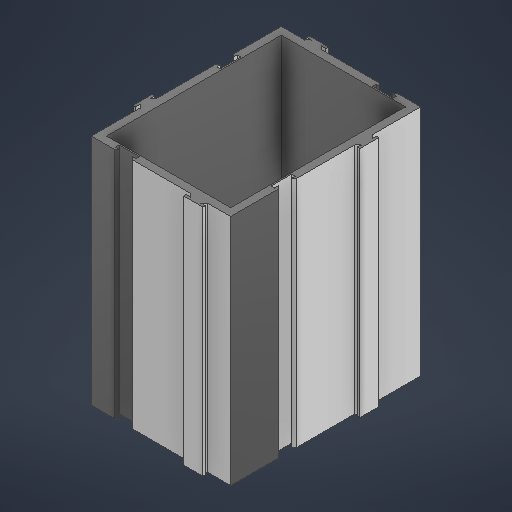
# Autodesk Inventor part: box
Saved by Autodesk Inventor 2027 (Build 310192060, 192F)
## iProperties
Created: 2026-06-08
Part Number: box
Material: Ogólny
Document SubType Name: Modeling
Designer: User
Density: 1 g/cm^3
Appearance: Domyślna
Author: User
Autodesk Inventor part; units mm, degrees
ref_plane "YZ Plane" through (0, 0, 0) normal (1, 0, 0) x (0, 1, 0)
ref_plane "XZ Plane" through (0, 0, 0) normal (0, 1, 0) x (-1, 0, 0)
ref_plane "XY Plane" through (0, 0, 0) normal (0, 0, 1) x (1, 0, 0)
sketch "Szkic1" plane through (0, 0, 0) normal (0, 1, 0) x (-1, 0, 0)
  line L0 (-27.5, -37.5) -> (27.5, -37.5)
  line L1 (27.5, -37.5) -> (27.5, 37.5)
  line L2 (27.5, 37.5) -> (-27.5, 37.5)
  line L3 (-27.5, 37.5) -> (-27.5, -37.5)
  line L4 (-27.5, -37.5) -> (27.5, 37.5) construction
  line L5 (27.5, -37.5) -> (-27.5, 37.5) construction
  line L6 (-24.5, -34.5) -> (24.5, -34.5)
  line L7 (24.5, -34.5) -> (24.5, 34.5)
  line L8 (24.5, 34.5) -> (-24.5, 34.5)
  line L9 (-24.5, 34.5) -> (-24.5, -34.5)
  line L10 (-24.5, -34.5) -> (24.5, 34.5) construction
  line L11 (24.5, -34.5) -> (-24.5, 34.5) construction
  line L12 (27.5, 37.5) -> (18.5607, 37.5)
  line L13 (27.5, 37.5) -> (36.4393, 37.5) construction
  line L14 (18.5607, 37.5) -> (17.5, 36.4393)
  line L15 (17.5, 36.4393) -> (19, 36.4393)
  line L16 (19, 36.4393) -> (19, 35.0393)
  line L17 (-27.5, 37.5) -> (-25.5, 37.5) construction
  line L18 (0, 34.5) -> (0, 37.5) construction
  line L19 (18.5607, 37.5) -> (32.6482, 37.5) construction
  line L20 (11.4393, 37.5) -> (29.6482, 37.5) construction
  line L21 (19, 35.0393) -> (15, 35.0393)
  line L22 (15, 35.0393) -> (15, 37.5) construction
  line L23 (11.4393, 37.5) -> (12.5, 36.4393)
  line L24 (12.5, 36.4393) -> (11, 36.4393)
  line L25 (11, 36.4393) -> (11, 35.0393)
  line L26 (11, 35.0393) -> (15, 35.0393)
  line L27 (-18.5607, 37.5) -> (-17.5, 36.4393) construction
  line L28 (-17.5, 36.4393) -> (-19, 36.4393) construction
  line L29 (-19, 35.0393) -> (-15, 35.0393) construction
  line L30 (-15, 35.0393) -> (-15, 37.5) construction
  line L31 (-11.4393, 37.5) -> (-12.5, 36.4393) construction
  line L32 (-11, 35.0393) -> (-15, 35.0393) construction
  line L33 (-11, 36.4393) -> (-11, 35.0393) construction
  line L34 (-12.5, 36.4393) -> (-11, 36.4393) construction
  line L35 (-19, 36.4393) -> (-19, 35.0393) construction
  line L36 (24.5, 0) -> (-24.5, 0) construction
  line L37 (27.5, 0) -> (24.5, 0) construction
  line L38 (18.5607, -37.5) -> (17.5, -36.4393) construction
  line L39 (17.5, -36.4393) -> (19, -36.4393) construction
  line L40 (19, -36.4393) -> (19, -35.0393) construction
  line L41 (19, -35.0393) -> (15, -35.0393) construction
  line L42 (15, -35.0393) -> (15, -37.5) construction
  line L43 (11.4393, -37.5) -> (12.5, -36.4393) construction
  line L44 (11, -35.0393) -> (15, -35.0393) construction
  line L45 (11, -36.4393) -> (11, -35.0393) construction
  line L46 (12.5, -36.4393) -> (11, -36.4393) construction
  line L47 (-11.4393, -37.5) -> (-12.5, -36.4393)
  line L48 (-12.5, -36.4393) -> (-11, -36.4393)
  line L49 (-15, -35.0393) -> (-15, -37.5) construction
  line L50 (-11, -35.0393) -> (-15, -35.0393)
  line L51 (-18.5607, -37.5) -> (-17.5, -36.4393)
  line L52 (-17.5, -36.4393) -> (-19, -36.4393)
  line L53 (-19, -35.0393) -> (-15, -35.0393)
  line L54 (-11, -36.4393) -> (-11, -35.0393)
  line L55 (-19, -36.4393) -> (-19, -35.0393)
  line L56 (27.5, 11.4393) -> (26.4393, 12.5) construction
  line L57 (26.4393, 12.5) -> (26.4393, 11) construction
  line L58 (26.4393, 11) -> (25.0393, 11) construction
  line L59 (25.0393, 11) -> (25.0393, 15) construction
  line L60 (25.0393, 15) -> (27.3, 15) construction
  line L61 (27.5, 18.5607) -> (26.4393, 17.5) construction
  line L62 (25.0393, 19) -> (25.0393, 15) construction
  line L63 (26.4393, 19) -> (25.0393, 19) construction
  line L64 (26.4393, 17.5) -> (26.4393, 19) construction
  line L65 (27.5, -11.4393) -> (26.4393, -12.5)
  line L66 (26.4393, -12.5) -> (26.4393, -11)
  line L67 (26.4393, -11) -> (25.0393, -11)
  line L68 (25.0393, -11) -> (25.0393, -15)
  line L69 (27.5, -18.5607) -> (26.4393, -17.5)
  line L70 (26.4393, -17.5) -> (26.4393, -19)
  line L71 (25.0393, -15) -> (27.3, -15) construction
  line L72 (25.0393, -19) -> (25.0393, -15)
  line L73 (26.4393, -19) -> (25.0393, -19)
  line L74 (-27.5, 11.4393) -> (-26.4393, 12.5)
  line L75 (-26.4393, 12.5) -> (-26.4393, 11)
  line L76 (-26.4393, 11) -> (-25.0393, 11)
  line L77 (-25.0393, 11) -> (-25.0393, 15)
  line L78 (-27.5, 18.5607) -> (-26.4393, 17.5)
  line L79 (-26.4393, 17.5) -> (-26.4393, 19)
  line L80 (-25.0393, 15) -> (-27.3, 15) construction
  line L81 (-25.0393, 19) -> (-25.0393, 15)
  line L82 (-26.4393, 19) -> (-25.0393, 19)
  line L83 (-27.5, -11.4393) -> (-26.4393, -12.5) construction
  line L84 (-26.4393, -12.5) -> (-26.4393, -11) construction
  line L85 (-26.4393, -11) -> (-25.0393, -11) construction
  line L86 (-25.0393, -11) -> (-25.0393, -15) construction
  line L87 (-25.0393, -15) -> (-27.3, -15) construction
  line L88 (-27.5, -18.5607) -> (-26.4393, -17.5) construction
  line L89 (-25.0393, -19) -> (-25.0393, -15) construction
  line L90 (-26.4393, -17.5) -> (-26.4393, -19) construction
  line L91 (-26.4393, -19) -> (-25.0393, -19) construction
  line L92 (-11.4393, 37.5) -> (-12.5, 38.5607)
  line L93 (-12.5, 38.5607) -> (-11, 38.5607)
  line L94 (-15, 39.9607) -> (-15, 37.5)
  line L95 (-11, 39.9607) -> (-15, 39.9607)
  line L96 (-18.5607, 37.5) -> (-17.5, 38.5607)
  line L97 (-17.5, 38.5607) -> (-19, 38.5607)
  line L98 (-19, 39.9607) -> (-15, 39.9607)
  line L99 (-11, 38.5607) -> (-11, 39.9607)
  line L100 (-19, 38.5607) -> (-19, 39.9607)
  line L101 (18.5607, -37.5) -> (17.5, -38.5607)
  line L102 (17.5, -38.5607) -> (19, -38.5607)
  line L103 (19, -38.5607) -> (19, -39.9607)
  line L104 (19, -39.9607) -> (15, -39.9607)
  line L105 (11, -39.9607) -> (15, -39.9607)
  line L106 (15, -39.9607) -> (15, -37.5) construction
  line L107 (11.4393, -37.5) -> (12.5, -38.5607)
  line L108 (11, -38.5607) -> (11, -39.9607)
  line L109 (12.5, -38.5607) -> (11, -38.5607)
  line L110 (27.5, 11.4393) -> (28.5607, 12.5)
  line L111 (28.5607, 12.5) -> (28.5607, 11)
  line L112 (28.5607, 11) -> (29.9607, 11)
  line L113 (29.9607, 11) -> (29.9607, 15)
  line L114 (27.5, 18.5607) -> (28.5607, 17.5)
  line L115 (28.5607, 17.5) -> (28.5607, 19)
  line L116 (29.9607, 15) -> (27.7, 15) construction
  line L117 (29.9607, 19) -> (29.9607, 15)
  line L118 (28.5607, 19) -> (29.9607, 19)
  line L119 (-28.5607, -19) -> (-29.9607, -19)
  line L120 (-28.5607, -17.5) -> (-28.5607, -19)
  line L121 (-27.5, -18.5607) -> (-28.5607, -17.5)
  line L122 (-29.9607, -11) -> (-29.9607, -15)
  line L123 (-29.9607, -15) -> (-27.7, -15) construction
  line L124 (-28.5607, -11) -> (-29.9607, -11)
  line L125 (-28.5607, -12.5) -> (-28.5607, -11)
  line L126 (-27.5, -11.4393) -> (-28.5607, -12.5)
  line L127 (-29.9607, -19) -> (-29.9607, -15)
  point P0 (0, 0)
  point P1 (-11.4393, 37.5)
  point P2 (-18.5607, 37.5)
  point P3 (-18.5607, -37.5)
  point P4 (-11.4393, -37.5)
  point P5 (11.4393, -37.5)
  point P6 (18.5607, -37.5)
  point P7 (0, 36)
  point P8 (15, 36.2697)
  point P9 (26, 0)
  point P10 (-15, 36.2697)
  point P11 (26.1697, 15)
  point P12 (26.1697, -15)
  point P13 (-26.1697, 15)
  point P14 (-26.1697, -15)
  point P15 (26.1697, -15)
  point P16 (-27.5, 11.4393)
  point P17 (-27.5, -11.4393)
  point P18 (-27.5, -18.5607)
  point P19 (27.5, -18.5607)
  point P20 (27.5, -11.4393)
  point P21 (-15, 38.7303)
  point P22 (28.8303, 15)
  point P23 (-28.8303, -15)
  point P24 (18.5607, -37.5)
  point P25 (11.4393, -37.5)
  point P26 (-11.4393, 37.5)
  dimension "d0" = 55
  dimension "d1" = 75
  dimension "d2" = 49
  dimension "d3" = 69
  dimension "d6" = 1.5
  dimension "d7" = 135
  dimension "d8" = 1.5
  dimension "d9" = 1.4
  dimension "d15" = 2
  dimension "d23" = 4
  dimension "d29" = 45
  dimension "d32" = 15
  dimension "d34" = 1.5
  dimension "d35" = 1.5
  dimension "d36" = 1.4
  dimension "d37" = 4
  dimension "d38" = 45
  dimension "d39" = 15
  dimension "d76" = 1.1303
  constraints: 256 end point, 102 symmetric about line, 15 midpoint, 10 parallel, 7 point on line, 4 horizontal, 4 perpendicular, 2 collinear, 2 vertical
  measures "d0" distance of L2.end L1.end
  measures "d1" distance of L1.end L0.end
  measures "d2" distance of L8.end L7.end
  measures "d3" distance of L7.end L6.end
  measures "d6" distance of L12.end L14.end
  measures "d7" angle of L14 L12
  measures "d8" distance of L14.end L15.end
  measures "d9" distance of L15.end L16.end
  measures "d15" distance of L2.end L17.end
  measures "d23" distance of L16.end L21.end
  measures "d29" angle of L24 L23
  measures "d32" distance from line of point (0, 36) L22
  measures "d34" distance of L56.start L56.end
  measures "d35" distance of L56.end L57.end
  measures "d36" distance of L57.end L58.end
  measures "d37" distance of L58.end L59.end
  measures "d38" angle of L64 L61
  measures "d39" vertical distance of point (26, 0) point (26.17, 15)
  measures "d76" distance of L68.end point (26.17, -15)
extrude "Wyciągnięcie proste1" add sketch "Szkic1" along normal blind 90 contours L3 L74 L75 L76 L77 L81 L82 L79 L78 L2 L23 L24 L25 L26 L21 L16 L15 L14 L1 L65 L66 L67 L68 L72 L73 L70 L69 L0 L47 L48 L54 L50 L53 L55 L52 L51 | L121 L120 L119 L127 L122 L124 L125 L126 L3 | L0 L101 L102 L103 L104 L105 L108 L109 L107 | L96 L97 L100 L98 L94 L2 | L94 L95 L99 L93 L92 L2 | L1 L114 L115 L118 L117 L113 L112 L111 L110
extrude "Wyciągnięcie proste2" add sketch "Szkic1" against normal blind 2 contours L3 L74 L75 L76 L77 L81 L82 L79 L78 L2 L23 L24 L25 L26 L21 L16 L15 L14 L1 L65 L66 L67 L68 L72 L73 L70 L69 L0 L47 L48 L54 L50 L53 L55 L52 L51 | L121 L120 L119 L127 L122 L124 L125 L126 L3 | L0 L101 L102 L103 L104 L105 L108 L109 L107 | L96 L97 L100 L98 L94 L2 | L94 L95 L99 L93 L92 L2 | L1 L114 L115 L118 L117 L113 L112 L111 L110 | L9 L8 L7 L6
offset faces "Rozmiar1" outward -0.2 faces at (-19, 28.6667, -39.494) (-17.8536, 28.6667, -38.2071) (-13.6667, 28.6667, -39.9607) (-11, 28.6667, -39.0273) (-11.7929, 28.6667, -37.8536) (-12, 28.6667, -38.5607) (-18.5, 28.6667, -38.5607) (-28.5607, 28.6667, 12) (-29.0273, 28.6667, 11) (-28.2071, 28.6667, 17.8536) (-29.494, 28.6667, 19) (-28.5607, 28.6667, 18.5) (-27.8536, 28.6667, 11.7929) (-29.9607, 28.6667, 13.6667) (16.3333, 59.3333, 39.9607) (19, 59.3333, 39.0273) (18.2071, 59.3333, 37.8536) (18, 59.3333, 38.5607) (11.5, 59.3333, 38.5607) (11, 59.3333, 39.494) (12.1464, 59.3333, 38.2071) (28.5607, 59.3333, -11.5) (29.494, 59.3333, -11) (29.9607, 59.3333, -16.3333) (29.0273, 59.3333, -19) (28.5607, 59.3333, -18)
equation "\"Offcenter\" = 15"
equation "\"width\" = 75"
equation "\"height\" = 55"
